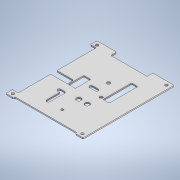
# Autodesk Inventor part: mainunitshield
Saved by Autodesk Inventor 2021 (Build 250183000, 183)
## iProperties
Created: 2022-12-06
Part Number: mainunitshield
Material: Generisch
Document SubType Name: Blech
Designer: WS
Density: 1 g/cm^3
Appearance: Vorgabe
Sheet Metal Rule: Standard_mm
Author: WS
Autodesk Inventor part; units mm, degrees
ref_plane "YZ Plane" through (0, 0, 0) normal (1, 0, 0) x (0, 1, 0)
ref_plane "XZ Plane" through (0, 0, 0) normal (0, 1, 0) x (-1, 0, 0)
ref_plane "XY Plane" through (0, 0, 0) normal (0, 0, 1) x (1, 0, 0)
sketch "Skizze1" plane through (0, 0, 0) normal (0, 1, 0) x (-1, 0, 0)
  line L0 (10, 0) -> (90, 0)
  line L1 (100, 0) -> (100, -116)
  line L2 (100, -116) -> (0, -116)
  line L3 (0, -116) -> (0, 0)
  line L4 (100, 0) -> (90, 0)
  line L5 (90, 0) -> (90, 2)
  line L6 (90, 2) -> (100, 2)
  line L7 (100, 2) -> (100, 0)
  line L8 (0, 0) -> (10, 0)
  line L9 (10, 0) -> (10, 2)
  line L10 (10, 2) -> (0, 2)
  line L11 (0, 2) -> (0, 0)
  dimension "d0" = 116
  dimension "d1" = 100
  dimension "d58" = 10
  dimension "d59" = 2
  dimension "d60" = 10
  dimension "d61" = 2
  constraints: 24 end point, 6 parallel, 3 horizontal, 3 perpendicular
  measures "d0" distance of L1.start L1.end
  measures "d1" distance between parallel lines of L3 L1
  measures "d58" distance of L5.end L6.end
  measures "d59" distance of L0.end L5.end
  measures "d60" distance of L10.end L9.end
  measures "d61" distance between parallel lines of L0 L10
extrude "Extrusion1" add sketch "Skizze1" along normal blind 1.6
sketch "Skizze2" plane through (0, 1.6, 0) normal (0, 1, 0) x (1, 0, 0)
  line L0 (0, 116) -> (-100, 116) projected
  line L1 (-100, 116) -> (-100, -2) projected
  point P0 (0, 0)
  point P1 (-95, 111)
  point P2 (-100, 0)
  dimension "d4" = 5
  dimension "d5" = 5
  measures "d4" distance from line of L0 point (-95, 111)
  measures "d5" distance from line of L1 point (-95, 111)
hole "Bohrung1" at (-95, 1.6, -111) direction (0, -1, 0) diameter 3.5 end through all
pattern_linear "Rechteckige Anordnung1" count 2 spacing 109 along (0, 0, 1) count 2 spacing 90 along (1, 0, 0) of "Bohrung1"
sketch "Skizze3" plane through (0, 1.6, 0) normal (0, 1, 0) x (1, 0, 0)
  line L0 (-98.5, 8.5) -> (-94.5, 8.5)
  line L1 (-94.5, 8.5) -> (-94.5, 105.5)
  line L2 (-94.5, 105.5) -> (-98.5, 105.5)
  line L3 (-98.5, 105.5) -> (-98.5, 8.5)
  line L4 (-100, 116) -> (-100, -2) projected
  line L5 (0, 116) -> (-100, 116) projected
  line L6 (-94, 50.5) -> (-73, 50.5)
  line L7 (-73, 50.5) -> (-73, 54.5)
  line L8 (-73, 54.5) -> (-94, 54.5)
  line L9 (-94, 54.5) -> (-94, 50.5)
  line L10 (-72.5, 110.5) -> (-29.5, 110.5)
  line L11 (-29.5, 110.5) -> (-29.5, 114.5)
  line L12 (-29.5, 114.5) -> (-72.5, 114.5)
  line L13 (-72.5, 114.5) -> (-72.5, 110.5)
  line L14 (-28, 56) -> (-24, 56)
  line L15 (-24, 56) -> (-24, 89)
  line L16 (-24, 89) -> (-28, 89)
  line L17 (-28, 89) -> (-28, 56)
  line L18 (0, 0) -> (0, 116) projected
  line L19 (-67.5, 50.5) -> (-62.5, 50.5)
  line L20 (-62.5, 50.5) -> (-62.5, 66.5)
  line L21 (-62.5, 66.5) -> (-67.5, 66.5)
  line L22 (-67.5, 66.5) -> (-67.5, 50.5)
  line L23 (-71, 48.5) -> (-96, 48.5)
  line L24 (-96, 48.5) -> (-96, 56.5)
  line L25 (-96, 56.5) -> (-71, 56.5)
  line L26 (-71, 56.5) -> (-71, 48.5)
  line L27 (-92.5, 107.5) -> (-92.5, 6.5)
  line L28 (-92.5, 6.5) -> (-100.5, 6.5)
  line L29 (-100.5, 6.5) -> (-100.5, 107.5)
  line L30 (-100.5, 107.5) -> (-92.5, 107.5)
  line L31 (-69.5, 48.5) -> (-60.5, 48.5)
  line L32 (-60.5, 48.5) -> (-60.5, 68.5)
  line L33 (-60.5, 68.5) -> (-69.5, 68.5)
  line L34 (-69.5, 68.5) -> (-69.5, 48.5)
  line L35 (-27.5, 108.5) -> (-74.5, 108.5)
  line L36 (-74.5, 108.5) -> (-74.5, 116.5)
  line L37 (-74.5, 116.5) -> (-27.5, 116.5)
  line L38 (-27.5, 116.5) -> (-27.5, 108.5)
  line L39 (-30, 54) -> (-22, 54)
  line L40 (-22, 54) -> (-22, 91)
  line L41 (-22, 91) -> (-30, 91)
  line L42 (-30, 91) -> (-30, 54)
  point P0 (-100, 0)
  point P1 (-27.5, 116)
  point P2 (-74.5, 116)
  point P3 (-92.5, 48.5)
  point P4 (-92.5, 56.5)
  point P5 (-100, 107.5)
  point P6 (-100, 6.5)
  dimension "d19" = 97
  dimension "d20" = 4
  dimension "d21" = 1.5
  dimension "d22" = 10.5
  dimension "d23" = 4
  dimension "d24" = 21
  dimension "d25" = 61.5
  dimension "d26" = 6
  dimension "d27" = 43
  dimension "d28" = 4
  dimension "d29" = 1.5
  dimension "d30" = 27.5
  dimension "d31" = 4
  dimension "d32" = 33
  dimension "d33" = 24
  dimension "d34" = 27
  dimension "d47" = 5
  dimension "d48" = 16
  dimension "d49" = 0
  dimension "d50" = 62.5
  dimension "d53" = 2
  dimension "d54" = 2
  dimension "d55" = 2
  dimension "d56" = 2
  dimension "d57" = 2
  constraints: 80 end point, 20 parallel, 10 perpendicular, 5 horizontal, 15 other
  measures "d19" distance of L2.end L0.start
  measures "d20" distance between parallel lines of L1 L3
  measures "d21" distance between parallel lines of L4 L3
  measures "d22" distance between parallel lines of L5 L2
  measures "d23" distance of L6.end L7.end
  measures "d24" distance of L6.start L6.end
  measures "d25" distance between parallel lines of L5 L8
  measures "d26" distance between parallel lines of L4 L9
  measures "d27" distance of L11.end L12.end
  measures "d28" distance of L10.end L11.end
  measures "d29" distance between parallel lines of L5 L12
  measures "d30" distance between parallel lines of L13 L4
  measures "d31" distance of L16.end L15.end
  measures "d32" distance of L15.end L14.end
  measures "d33" distance between parallel lines of L18 L15
  measures "d34" distance between parallel lines of L5 L16
  measures "d47" distance of L21.end L20.end
  measures "d48" distance of L20.end L19.end
  measures "d49" distance between parallel lines of L6 L19
  measures "d50" distance between parallel lines of L18 L20
  measures "d53" distance between parallel lines of L6 L23
  measures "d54" distance between parallel lines of L1 L27
  measures "d55" distance between parallel lines of L22 L34
  measures "d56" distance between parallel lines of L10 L35
  measures "d57" distance between parallel lines of L17 L42
extrude "Extrusion2" cut sketch "Skizze3" against normal through all contours L3 L2 L1 L25 L24 L23 L0 | L0 L1 L23 L27 L28 L4 L30 L25 L2 L3 | L23 L24 L25 L1 | L1 L25 L27 L8 L9 L6 L23 | L27 L6 L7 L8 L25 L26 L23 | L5 L38 L35 L36 | L27 L8 L7 L6 | L6 L9 L8 L27 | L13 L12 L11 L10 | L17 L16 L15 L14 | L22 L21 L20 L19 | L34 L33 L32 L31 | L42 L41 L40 L39
fillet "Rundung1" radius 1 28 edges at (-100, 0.8, 2) (-100, 0.8, -116) (-74.5, 0.8, -116) (-74.5, 0.8, -108.5) (-69.5, 0.8, -68.5) (-60.5, 0.8, -68.5) (-60.5, 0.8, -48.5) (-69.5, 0.8, -48.5) (-71, 0.8, -56.5) (-71, 0.8, -48.5) (-92.5, 0.8, -56.5) (-92.5, 0.8, -48.5) (-90, 0.8, 0) (-90, 0.8, 2) (-92.5, 0.8, -6.5) (-100, 0.8, -6.5) (-10, 0.8, 2) (-10, 0.8, 0) (0, 0.8, 2) (-22, 0.8, -54) (-30, 0.8, -54) (-30, 0.8, -91) (-22, 0.8, -91) (-27.5, 0.8, -108.5) (-27.5, 0.8, -116) (0, 0.8, -116) (-92.5, 0.8, -107.5) (-100, 0.8, -107.5)
sketch "Skizze4" plane through (0, 1.6, 0) normal (0, 1, 0) x (1, 0, 0)
  circle A0 centre (-45, 76) radius 2
  line L0 (-1, 116) -> (-26.5, 116) projected
  line L1 (0, -1) -> (0, 115) projected
  circle A1 centre (-33.5, 55) radius 2
  line L2 (-52, 60.5) -> (-45, 60.5) construction
  line L3 (-52, 58.5) -> (-45, 58.5)
  line L4 (-45, 62.5) -> (-52, 62.5)
  arc A2 (-52, 62.5) -> (-52, 58.5) centre (-52, 60.5) ccw
  arc A3 (-45, 58.5) -> (-45, 62.5) centre (-45, 60.5) ccw
  line L5 (-75.5, 116) -> (-99, 116) projected
  line L6 (-100, 115) -> (-100, 108.5) projected
  circle A4 centre (-46, 38.5) radius 3
  circle A5 centre (-35, 38.5) radius 3
  line L7 (-9, -2) -> (-1, -2) projected
  line L8 (-64, 17) -> (-64, 36) construction
  line L9 (-62, 17) -> (-62, 36)
  line L10 (-66, 36) -> (-66, 17)
  arc A6 (-66, 17) -> (-62, 17) centre (-64, 17) ccw
  arc A7 (-62, 36) -> (-66, 36) centre (-64, 36) ccw
  line L11 (-100, 5.5) -> (-100, -1) projected
  line L12 (-64, 36) -> (-69, 36) construction
  line L13 (-64, 38) -> (-69, 38)
  line L14 (-69, 34) -> (-64, 34)
  arc A8 (-64, 34) -> (-64, 38) centre (-64, 36) ccw
  arc A9 (-69, 38) -> (-69, 34) centre (-69, 36) ccw
  circle A10 centre (-45, 16) radius 1.5
  point P0 (0, 0)
  point P1 (-48.5, 60.5)
  point P2 (-64, 26.5)
  point P3 (-66.5, 36)
  dimension "d63" = 4
  dimension "d64" = 40
  dimension "d65" = 45
  dimension "d66" = 4
  dimension "d67" = 33.5
  dimension "d68" = 61
  dimension "d69" = 7
  dimension "d70" = 4
  dimension "d71" = 55.5
  dimension "d72" = 48
  dimension "d73" = 6
  dimension "d74" = 6
  dimension "d75" = 11
  dimension "d76" = 0
  dimension "d77" = 35
  dimension "d79" = 77.5
  dimension "d80" = 19
  dimension "d81" = 4
  dimension "d82" = 36
  dimension "d83" = 80
  dimension "d84" = 5
  dimension "d85" = 4
  dimension "d86" = 3
  dimension "d87" = 100
  dimension "d88" = 45
  constraints: 24 end point, 12 point on circle, 12 tangent, 11 centre point, 3 midpoint, 3 parallel, 1 horizontal, 1 perpendicular, 1 vertical
  measures "d63" diameter of A0
  measures "d64" distance from line of L0 A0.centre
  measures "d65" distance from line of L1 A0.centre
  measures "d66" diameter of A1
  measures "d67" distance from line of L1 A1.centre
  measures "d68" distance from line of L0 A1.centre
  measures "d69" distance of L2.start L2.end
  measures "d70" diameter of A3
  measures "d71" distance between parallel lines of L5 L2
  measures "d72" distance from line of L6 L2.start
  measures "d73" diameter of A4
  measures "d74" diameter of A5
  measures "d75" distance of A4.centre A5.centre
  measures "d76" vertical distance of A4.centre A5.centre
  measures "d77" distance from line of L1 A5.centre
  measures "d79" distance from line of L0 A5.centre
  measures "d80" distance of L8.start L8.end
  measures "d81" diameter of A7
  measures "d82" distance between parallel lines of L8 L11
  measures "d83" distance from line of L5 L8.end
  measures "d84" distance of L8.end L12.end
  measures "d85" diameter of A9
  measures "d86" diameter of A10
  measures "d87" distance from line of L0 A10.centre
  measures "d88" distance from line of L1 A10.centre
extrude "Ausklinkung1" cut sketch "Skizze4" against normal blind 2
equation "\"Biegeradius\" = Stärke"
equation "\"BreiteBiegungsfreistellung\" = Stärke"
equation "\"TiefeBiegungsfreistellung\" = 0.5 * Stärke"
equation "\"GrößeEckenfreistellung\" = 4 * Stärke"
equation "\"MinimalRest\" = 2 * Stärke"
equation "\"Übergangsradius\" = Biegeradius"
equation "\"JacobiRadiusGröße\" = Biegeradius"
equation "\"Abstandsgröße\" = Stärke"
equation "\"d89\" = Stärke"
equation "\"Stärke\" = 1.5"
